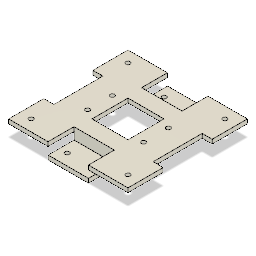
底盘 (Autodesk Fusion 360 design; units mm, degrees)
Autodesk Fusion 360 part; units mm, degrees
sketch "Sketch1" plane through (0, 0, 0) normal (0, 1, 0) x (1, 0, 0)
  line L0 (41.5, 41.5) -> (-41.5, 41.5)
  line L1 (-41.5, -41.5) -> (41.5, -41.5)
  line L2 (-41.5, 41.5) -> (41.5, -41.5) construction
  line L3 (41.5, 41.5) -> (41.5, 17)
  line L4 (41.5, 17) -> (34.5, 17)
  line L5 (-41.5, 41.5) -> (-41.5, 17)
  line L6 (-41.5, 17) -> (-34.5, 17)
  line L7 (-41.5, -17) -> (-34.5, -17)
  line L8 (41.5, -17) -> (34.5, -17)
  line L9 (-34.5, 17) -> (-34.5, -17)
  line L10 (34.5, 17) -> (34.5, -17)
  line L11 (-41.5, 41.5) -> (-41.5, 17)
  line L12 (-41.5, -17) -> (-41.5, -41.5)
  line L13 (-41.5, -41.5) -> (-41.5, -17)
  line L14 (-41.5, 17) -> (-41.5, 41.5)
  line L15 (41.5, -41.5) -> (41.5, -17)
  line L16 (41.5, 17) -> (41.5, 41.5)
  line L17 (41.5, 41.5) -> (41.5, 17)
  line L18 (41.5, -17) -> (41.5, -41.5)
  line L19 (-34.5, 17) -> (-34.5, 8.6)
  line L20 (-34.5, -17) -> (-34.5, -8.6)
  line L21 (34.5, 17) -> (34.5, 8.6)
  line L22 (34.5, -17) -> (34.5, -8.6)
  line L23 (-41.5, 41.5) -> (-33.655, 41.5)
  line L24 (-33.655, 41.5) -> (-41.5, 41.5)
  line L25 (-41.5, 41.5) -> (-41.5, 33.655)
  circle A0 centre (-33.655, 33.655) radius 1.55
  circle A1 centre (33.655, 33.655) radius 1.55
  circle A2 centre (-33.655, -33.655) radius 1.55
  circle A3 centre (33.655, -33.655) radius 1.55
  line L26 (11, 11) -> (-11, -11) construction
  line L27 (-11, 11) -> (11, -11) construction
  line L28 (12.5, -12.5) -> (-12.5, -12.5)
  line L29 (-12.5, -12.5) -> (-12.5, 12.5)
  line L30 (-12.5, 12.5) -> (12.5, 12.5)
  line L31 (12.5, 12.5) -> (12.5, -12.5)
  line L32 (12.5, -12.5) -> (-12.5, 12.5) construction
  line L33 (-12.5, -12.5) -> (12.5, 12.5) construction
  line L34 (-41.5, 41.5) -> (-14.05, 41.5)
  line L35 (-14.05, 41.5) -> (-8.5, 41.5)
  circle A4 centre (-8.5, 33.655) radius 1.55
  circle A5 centre (8.5, 33.655) radius 1.55
  line L36 (-14.05, 41.5) -> (-14.05, 23.5)
  line L37 (-14.05, 23.5) -> (14.05, 23.5)
  line L38 (14.05, 23.5) -> (14.05, 41.5)
  line L39 (-14.05, -23.5) -> (14.05, -23.5)
  circle A6 centre (8.5, -33.655) radius 1.55
  circle A7 centre (-8.5, -33.655) radius 1.55
  line L40 (-14.05, -41.5) -> (-14.05, -23.5)
  line L41 (14.05, -23.5) -> (14.05, -41.5)
  circle A8 centre (-19.5, 8.6) radius 1.55
  circle A9 centre (-19.5, -8.6) radius 1.55
  circle A10 centre (19.5, 8.6) radius 1.55
  circle A11 centre (19.5, -8.6) radius 1.55
  point P0 (-19.5, 8.6)
  point P1 (19.5, 8.6)
  dimension "d1" = 83
  dimension "d2" = 83
  dimension "d31" = 27.45
  dimension "d32" = 5.55
  dimension "d33" = 7.845
  dimension "d34" = 17
  dimension "d35" = 3.1
  dimension "d36" = 3.1
  dimension "d37" = 18
  dimension "d39" = 18
  dimension "d40" = 3.1
  constraint perpendicular L0 L11
  constraint parallel L0 L1
  constraint parallel L11 L15
  constraint horizontal L0
  constraint perpendicular L0 L3
  constraint perpendicular L4 L15
  constraint perpendicular L7 L9
  constraint perpendicular L8 L10
  constraint collinear L11 L12
  constraint collinear L13 L14
  constraint collinear L15 L16
  constraint collinear L17 L18
  constraint perpendicular L6 L19
  constraint perpendicular L7 L20
  constraint perpendicular L4 L21
  constraint perpendicular L8 L22
  constraint perpendicular L5 L23
  constraint horizontal L24
  constraint vertical L25
  constraint coincident L26 origin
  constraint coincident L27 origin
  constraint midpoint L2 origin
  constraint perpendicular L28 L29
  constraint parallel L28 L30
  constraint parallel L29 L31
  constraint horizontal L28
  constraint coincident L32 origin
  constraint coincident L33 origin
  constraint perpendicular L5 L34
  constraint parallel L0 L35
  constraint perpendicular L34 L36
  constraint perpendicular L36 L37
  constraint perpendicular L0 L38
  constraint coincident P0 A8.centre
  measures "d1" distance of L1.start L1.end
  measures "d2" distance of L0.end L1.start
  measures "d31" distance of L0.end L34.end
  measures "d32" distance of L34.end L35.end
  measures "d33" distance of L35.end A4.centre
  measures "d34" distance of A4.centre A5.centre
  measures "d35" diameter of A4
  measures "d36" diameter of A5
  measures "d37" distance of L34.end L36.end
  measures "d39" distance of L37.end L38.end
  measures "d40" diameter of A8
extrude "Extrude4" add sketch "Sketch1" along normal blind 8 contours L0 L1 L3 L4 L5 L6 L7 L8 L9 L10 L11 L12 L13 L14 L15 L16 L17 L18 L19 L20 L21 L22 L23 L24 L25 L34 L36 L37 L38 L39 L40 L41 makes body 1
sketch "Sketch2" plane through (0, 8, 0) normal (0, 1, 0) x (-1, 0, 0)
  circle A0 centre (-19.5, -8.6) radius 1.55
  circle A1 centre (33.655, 33.655) radius 1.55
  circle A2 centre (19.5, -8.6) radius 1.55
  circle A3 centre (19.5, 8.6) radius 1.55
  circle A4 centre (-19.5, 8.6) radius 1.55
  line L0 (12.5, -12.5) -> (-12.5, -12.5)
  line L1 (-12.5, -12.5) -> (-12.5, 12.5)
  line L2 (-12.5, 12.5) -> (12.5, 12.5)
  line L3 (12.5, 12.5) -> (12.5, -12.5)
  circle A5 centre (-33.655, -33.655) radius 1.55
  circle A6 centre (33.655, -33.655) radius 1.55
  circle A7 centre (-33.655, 33.655) radius 1.55
  line L4 (41.5, 41.5) -> (14.05, 41.5)
  line L5 (14.05, 41.5) -> (14.05, 23.5)
  line L6 (14.05, 23.5) -> (-14.05, 23.5)
  line L7 (-14.05, 23.5) -> (-14.05, 41.5)
  line L8 (-14.05, 41.5) -> (-41.5, 41.5)
  line L9 (-41.5, 41.5) -> (-41.5, 17)
  line L10 (-41.5, 17) -> (-34.5, 17)
  line L11 (-34.5, 17) -> (-34.5, -17)
  line L12 (-34.5, -17) -> (-41.5, -17)
  line L13 (-41.5, -17) -> (-41.5, -41.5)
  line L14 (-41.5, -41.5) -> (-14.05, -41.5)
  line L15 (-14.05, -41.5) -> (-14.05, -23.5)
  line L16 (-14.05, -23.5) -> (14.05, -23.5)
  line L17 (14.05, -23.5) -> (14.05, -41.5)
  line L18 (14.05, -41.5) -> (41.5, -41.5)
  line L19 (41.5, -41.5) -> (41.5, -17)
  line L20 (41.5, -17) -> (34.5, -17)
  line L21 (34.5, -17) -> (34.5, 17)
  line L22 (34.5, 17) -> (41.5, 17)
  line L23 (41.5, 17) -> (41.5, 41.5)
extrude "Extrude5" cut sketch "Sketch2" against normal blind 3 keep common part bodies 1
sketch "Sketch3" plane through (0, 0, 23.5) normal (0, 0, 1) x (1, 0, 0)
  line L0 (-14.05, 5) -> (14.05, 5)
  line L1 (14.05, 5) -> (14.05, 8)
  line L2 (14.05, 8) -> (-14.05, 8)
  line L3 (-14.05, 8) -> (-14.05, 5)
  line L4 (-14.05, 8) -> (-14.05, 0)
  line L5 (-14.05, 0) -> (14.05, 0)
  line L6 (14.05, 0) -> (14.05, 8)
  line L7 (14.05, 8) -> (-14.05, 8)
  line L8 (-14.05, 8) -> (-14.05, 0)
  line L9 (-14.05, 0) -> (14.05, 0)
  dimension "d47" = 28.1
  constraint coincident L2.end L3.start
  constraint perpendicular L0 L4
  constraint perpendicular L4 L5
  constraint perpendicular L6 L7
  constraint parallel L6 L8
  constraint parallel L7 L9
  constraint coincident L1.end L2.start
  measures "d47" distance of L4.end L5.end
extrude "Extrude6" add sketch "Sketch3" against normal blind 3 contours L0 L4 L5 L6 L8 L9 bodies 1
extrude "Extrude7" add sketch "Sketch1" against normal blind 3 separate body contours L1 L39 L40 L41 makes body 2
sketch "Sketch4" plane through (0, 0, 23.5) normal (0, 0, 1) x (1, 0, 0)
  line L0 (14.05, 5) -> (14.05, 8)
  line L1 (14.05, 8) -> (-14.05, 8)
  line L2 (-14.05, 8) -> (-14.05, 5)
  line L3 (-14.05, 5) -> (-14.05, 0)
  line L4 (-14.05, 0) -> (14.05, 0)
  line L5 (14.05, 0) -> (14.05, 5)
  line L6 (-14.05, 0) -> (-14.05, -3)
  line L7 (-14.05, -3) -> (14.05, -3)
  line L8 (-14.05, 0) -> (14.05, 0)
  line L9 (14.05, 0) -> (14.05, -3)
  line L10 (14.05, -3) -> (-14.05, -3)
  line L11 (-14.05, -3) -> (-14.05, 0)
  dimension "d52" = 3
  dimension "d53" = 28.1
  constraint coincident L3.end L4.start
  constraint perpendicular L4 L6
  constraint perpendicular L6 L7
  constraint horizontal L8
  constraint vertical L9
  constraint horizontal L10
  constraint vertical L11
  measures "d52" distance of L3.end L6.end
  measures "d53" distance of L6.end L7.end
extrude "Extrude8" add sketch "Sketch4" against normal blind 3 contours L4 L6 L7 L8 L9 L10 L11 bodies 1 2
sketch "Sketch5" plane through (0, 0, -23.5) normal (0, 0, -1) x (-1, 0, 0)
  line L0 (-14.05, 5) -> (14.05, 5)
  line L1 (14.05, 5) -> (14.05, 8)
  line L2 (14.05, 8) -> (-14.05, 8)
  line L3 (-14.05, 8) -> (-14.05, 5)
  line L4 (-14.05, 5) -> (-14.05, -3)
  line L5 (-14.05, -3) -> (14.05, -3)
  line L6 (14.05, -3) -> (-14.05, -3)
  line L7 (-14.05, -3) -> (-14.05, 5)
  line L8 (-14.05, 5) -> (14.05, 5)
  line L9 (14.05, 5) -> (14.05, -3)
  dimension "d56" = 8
  dimension "d57" = 28.1
  constraint coincident L0.start L3.end
  constraint perpendicular L0 L4
  constraint perpendicular L4 L5
  constraint perpendicular L6 L7
  constraint parallel L6 L8
  constraint parallel L7 L9
  measures "d56" distance of L0.start L4.end
  measures "d57" distance of L4.end L5.end
extrude "Extrude9" add sketch "Sketch5" against normal blind 3 contours L0 L4 L5 L6 L7 L8 L9 bodies 1
extrude "Extrude10" add sketch "Sketch1" against normal blind 3 contours L0 L35 L36 L37 L38 bodies 1
